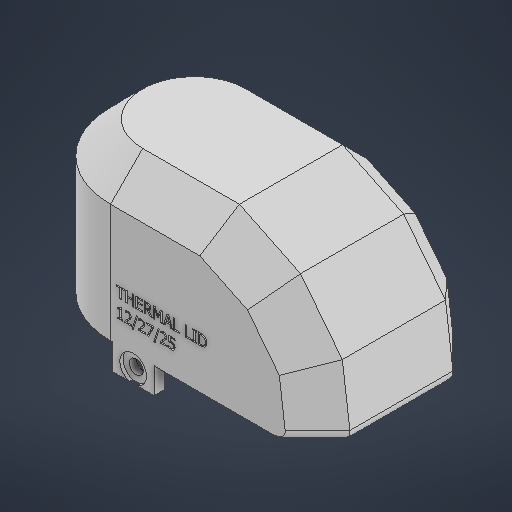
# Autodesk Inventor part: Thermal Lid
Saved by Autodesk Inventor 2026.2 (Build 302298000, 298)
## iProperties
Created: 2025-12-29
Part Number: Thermal Lid
Material: Generic
Document SubType Name: Modeling
Designer: mumin
Density: 1 g/cm^3
Appearance: Default
Author: mumin
Autodesk Inventor part; units mm, degrees
ref_plane "YZ Plane" through (0, 0, 0) normal (1, 0, 0) x (0, 1, 0)
ref_plane "XZ Plane" through (0, 0, 0) normal (0, 1, 0) x (-1, 0, 0)
ref_plane "XY Plane" through (0, 0, 0) normal (0, 0, 1) x (1, 0, 0)
sketch "Sketch1" plane through (0, 0, 0) normal (0, 0, 1) x (1, 0, 0)
  line L0 (0, 0) -> (0, 70)
  line L1 (0, 70) -> (84, 70)
  line L2 (84, 70) -> (112.4484, 56.2384)
  line L3 (112.4484, 56.2384) -> (131.9046, 31.3356)
  line L4 (131.9046, 31.3356) -> (136, 0)
  line L5 (-27.2, 0) -> (163.2, 0) projected
  line L6 (0, 0) -> (136, 0)
  dimension "d0" = 70
  dimension "d1" = 84
  dimension "d2" = 52
  dimension "d3" = 52
  constraints: 12 end point, 2 equal length, 1 collinear, 1 perpendicular, 1 point on line, 1 vertical
  measures "d0" distance of L0.start L0.end
  measures "d1" distance of L0.end L1.end
  measures "d2" horizontal distance of L1.end L4.end
  measures "d3" angle of L5 L3
extrude "Bilateral Extrude" add sketch "Sketch1" along normal mid plane 78
sketch "Sketch2" plane through (0, 70, -39) normal (0, 1, 0) x (1, 0, 0)
  line L0 (0, -39) -> (136, -39)
  line L1 (136, 0) -> (136, -78) projected
  line L2 (84, -78) -> (0, -78) projected
  arc A0 (39, 0) -> (39, -78) centre (39, -39) ccw
  line L3 (39, -39) -> (39, 0) construction
  line L4 (39, -39) -> (39, -78) construction
  line L5 (0, 0) -> (0, -78) projected
  line L6 (39, 0) -> (0, 0)
  line L7 (0, -78) -> (39, -78)
  dimension "d6" = 180
  constraints: 10 end point, 2 perpendicular, 2 point on circle, 2 point on line, 2 tangent, 1 centre point, 1 collinear, 1 midpoint
  measures "d6" angle of L3 L4
extrude "Rounded Front" cut sketch "Sketch2" against normal through all
shell "Shell1" thickness 5 removed faces 1 at (103.6667, 0, 13)
chamfer "Inside Chamfer" distance 12 angle 45 9 edges at (129.0406, 14.6667, 34) (118.174, 40.7886, 34) (96.0392, 58.6219, 34) (96.0392, 58.6219, -34) (118.174, 40.7886, -34) (129.0406, 14.6667, -34) (60.9271, 65, 34) (5, 65, 0) (60.9271, 65, -34)
chamfer "Outside Chamfer" distance 15 angle 45 9 edges at (61.5, 70, 39) (0, 70, 0) (61.5, 70, -39) (98.2242, 63.1192, 39) (98.2242, 63.1192, -39) (122.1765, 43.787, -39) (122.1765, 43.787, 39) (133.9523, 15.6678, 39) (133.9523, 15.6678, -39)
sketch "Sketch3" plane through (39, 0, 0) normal (0, -1, 0) x (1, 0, 0)
  line L0 (-39, -3.8185) -> (-39, 59.6275) construction
  line L1 (0.8, 39) -> (20.3, 39)
  line L2 (20.3, 39) -> (20.3, 34.2)
  line L3 (20.3, 34.2) -> (0.8, 34.2)
  line L4 (0.8, 34.2) -> (0.8, 39)
  line L5 (0, 39) -> (81.8724, 39) construction
  arc A0 (0, 39) -> (0, -39) centre (0, 0) ccw construction
  point P0 (-39, 0)
  point P1 (10.55, 39)
  dimension "d16" = 19.5
  dimension "d17" = 4.8
  dimension "d18" = 49.55
  constraints: 10 end point, 2 parallel, 1 horizontal, 1 midpoint, 1 perpendicular, 1 point on line, 1 tangent, 1 vertical
  measures "d16" distance of L2.end L3.end
  measures "d17" distance of L1.end L2.end
  measures "d18" distance from line of point (10.55, 39) L0
extrude "Alignment Tab" add sketch "Sketch3" along normal blind 12
sketch "Sketch4" plane through (0, 0, 39) normal (0, 0, 1) x (1, 0, 0)
  line L0 (49.55, -12) -> (49.55, 3)
  line L1 (59.3, -12) -> (39.8, -12) projected
  point P0 (0, 0)
  point P1 (49.55, -6)
  dimension "d28" = 15
  dimension "d29" = 6
  constraints: 2 end point, 1 point on line, 1 vertical
  measures "d28" distance of L0.start L0.end
  measures "d29" distance from line of L1 point (49.55, -6)
hole "Hole1" at (49.55, -6, 39) direction (0, 0, -1) diameter 6.5 depth 4.8 tip angle 118 counterbore diameter 12.5 counterbore depth 1.5
mirror "Mirror1" about plane through (0, 0, 0) normal (0, 0, 1) of "Alignment Tab", "Hole1"
sketch "Sketch6" plane through (0, 0, 39) normal (0, 0, 1) x (1, 0, 0)
  line L0 (41.5809, 23.9348) -> (84.0039, 23.9348) construction
  line L1 (84.0039, 23.9348) -> (84.0039, 9.6166) construction
  line L2 (84.0039, 9.6166) -> (41.5809, 9.6166) construction
  line L3 (41.5809, 9.6166) -> (41.5809, 23.9348) construction
  line L4 (43.2543, 18.9348) -> (43.2543, 23.3433)
  line L5 (43.2543, 23.3433) -> (41.5769, 23.3433)
  line L6 (41.5769, 23.3433) -> (41.5769, 23.9348)
  line L7 (41.5769, 23.9348) -> (45.5963, 23.9348)
  line L8 (45.5963, 23.9348) -> (45.5963, 23.3433)
  line L9 (45.5963, 23.3433) -> (43.9188, 23.3433)
  line L10 (43.9188, 23.3433) -> (43.9188, 18.9348)
  line L11 (43.9188, 18.9348) -> (43.2543, 18.9348)
  line L12 (49.7333, 18.9348) -> (49.0688, 18.9348)
  line L13 (49.0688, 18.9348) -> (49.0688, 21.3822)
  line L14 (49.0688, 21.3822) -> (46.7673, 21.3822)
  line L15 (46.7673, 21.3822) -> (46.7673, 18.9348)
  line L16 (46.7673, 18.9348) -> (46.1028, 18.9348)
  line L17 (46.1028, 18.9348) -> (46.1028, 23.9348)
  line L18 (46.1028, 23.9348) -> (46.7673, 23.9348)
  line L19 (46.7673, 23.9348) -> (46.7673, 21.9737)
  line L20 (46.7673, 21.9737) -> (49.0688, 21.9737)
  line L21 (49.0688, 21.9737) -> (49.0688, 23.9348)
  line L22 (49.0688, 23.9348) -> (49.7333, 23.9348)
  line L23 (49.7333, 23.9348) -> (49.7333, 18.9348)
  line L24 (50.7462, 18.9348) -> (50.7462, 23.9348)
  line L25 (50.7462, 23.9348) -> (53.8743, 23.9348)
  line L26 (53.8743, 23.9348) -> (53.8743, 23.3433)
  line L27 (53.8743, 23.3433) -> (51.4107, 23.3433)
  line L28 (51.4107, 23.3433) -> (51.4107, 21.9737)
  line L29 (51.4107, 21.9737) -> (53.7081, 21.9737)
  line L30 (53.7081, 21.9737) -> (53.7081, 21.3822)
  line L31 (53.7081, 21.3822) -> (51.4107, 21.3822)
  line L32 (51.4107, 21.3822) -> (51.4107, 19.5264)
  line L33 (51.4107, 19.5264) -> (53.8743, 19.5264)
  line L34 (53.8743, 19.5264) -> (53.8743, 18.9348)
  line L35 (53.8743, 18.9348) -> (50.7462, 18.9348)
  line L36 (58.4731, 18.9348) -> (57.6101, 18.9348)
  line L37 (57.6101, 18.9348) -> (56.0299, 20.9243)
  line L38 (56.0299, 20.9243) -> (55.2681, 20.9243)
  line L39 (55.2681, 20.9243) -> (55.2681, 18.9348)
  line L40 (55.2681, 18.9348) -> (54.6036, 18.9348)
  line L41 (54.6036, 18.9348) -> (54.6036, 23.9348)
  line L42 (54.6036, 23.9348) -> (55.8921, 23.9348)
  spline S0 degree 2 poles (55.8921, 23.9348) (56.3216, 23.9348) (56.901, 23.8416) (57.1644, 23.6715) knots 0 0 0 1 2 2 2
  spline S1 degree 2 poles (57.1644, 23.6715) (57.4278, 23.5013) (57.7316, 22.9705) (57.7316, 22.5775) knots 0 0 0 1 2 2 2
  spline S2 degree 2 poles (57.7316, 22.5775) (57.7316, 22.0305) (57.1725, 21.289) (56.6944, 21.1107) knots 0 0 0 1 2 2 2
  line L43 (56.6944, 21.1107) -> (58.4731, 18.9348)
  spline S3 degree 2 poles (57.0388, 22.5248) (57.0388, 22.7436) (56.8848, 23.0799) (56.7227, 23.1893) knots 0 0 0 1 2 2 2
  spline S4 degree 2 poles (56.7227, 23.1893) (56.5809, 23.2825) (56.2041, 23.3595) (55.9286, 23.3595) knots 0 0 0 1 2 2 2
  line L44 (55.9286, 23.3595) -> (55.2681, 23.3595)
  line L45 (55.2681, 23.3595) -> (55.2681, 21.4794)
  line L46 (55.2681, 21.4794) -> (55.8516, 21.4794)
  spline S5 degree 2 poles (55.8516, 21.4794) (56.1393, 21.4794) (56.5971, 21.5807) (56.7551, 21.7387) knots 0 0 0 1 2 2 2
  spline S6 degree 2 poles (56.7551, 21.7387) (56.901, 21.8765) (57.0388, 22.2655) (57.0388, 22.5248) knots 0 0 0 1 2 2 2
  line L47 (63.1571, 18.9348) -> (62.4926, 18.9348)
  line L48 (62.4926, 18.9348) -> (62.4926, 23.242)
  line L49 (62.4926, 23.242) -> (61.1879, 20.3125)
  line L50 (61.1879, 20.3125) -> (60.7827, 20.3125)
  line L51 (60.7827, 20.3125) -> (59.4902, 23.242)
  line L52 (59.4902, 23.242) -> (59.4902, 18.9348)
  line L53 (59.4902, 18.9348) -> (58.8702, 18.9348)
  line L54 (58.8702, 18.9348) -> (58.8702, 23.9348)
  line L55 (58.8702, 23.9348) -> (59.7778, 23.9348)
  line L56 (59.7778, 23.9348) -> (61.0258, 21.1512)
  line L57 (61.0258, 21.1512) -> (62.2333, 23.9348)
  line L58 (62.2333, 23.9348) -> (63.1571, 23.9348)
  line L59 (63.1571, 23.9348) -> (63.1571, 18.9348)
  line L60 (63.6312, 18.9348) -> (65.3167, 23.9348)
  line L61 (65.3167, 23.9348) -> (66.1352, 23.9348)
  line L62 (66.1352, 23.9348) -> (67.8208, 18.9348)
  line L63 (67.8208, 18.9348) -> (67.1198, 18.9348)
  line L64 (67.1198, 18.9348) -> (66.666, 20.3327)
  line L65 (66.666, 20.3327) -> (64.7576, 20.3327)
  line L66 (64.7576, 20.3327) -> (64.3038, 18.9348)
  line L67 (64.3038, 18.9348) -> (63.6312, 18.9348)
  line L68 (66.4837, 20.9) -> (65.7098, 23.2541)
  line L69 (65.7098, 23.2541) -> (64.9399, 20.9)
  line L70 (64.9399, 20.9) -> (66.4837, 20.9)
  line L71 (71.1919, 18.9348) -> (68.2949, 18.9348)
  line L72 (68.2949, 18.9348) -> (68.2949, 23.9348)
  line L73 (68.2949, 23.9348) -> (68.9594, 23.9348)
  line L74 (68.9594, 23.9348) -> (68.9594, 19.5264)
  line L75 (68.9594, 19.5264) -> (71.1919, 19.5264)
  line L76 (71.1919, 19.5264) -> (71.1919, 18.9348)
  line L77 (76.7592, 18.9348) -> (73.8621, 18.9348)
  line L78 (73.8621, 18.9348) -> (73.8621, 23.9348)
  line L79 (73.8621, 23.9348) -> (74.5266, 23.9348)
  line L80 (74.5266, 23.9348) -> (74.5266, 19.5264)
  line L81 (74.5266, 19.5264) -> (76.7592, 19.5264)
  line L82 (76.7592, 19.5264) -> (76.7592, 18.9348)
  line L83 (79.0242, 18.9348) -> (77.0874, 18.9348)
  line L84 (77.0874, 18.9348) -> (77.0874, 19.4454)
  line L85 (77.0874, 19.4454) -> (77.7235, 19.4454)
  line L86 (77.7235, 19.4454) -> (77.7235, 23.4243)
  line L87 (77.7235, 23.4243) -> (77.0874, 23.4243)
  line L88 (77.0874, 23.4243) -> (77.0874, 23.9348)
  line L89 (77.0874, 23.9348) -> (79.0242, 23.9348)
  line L90 (79.0242, 23.9348) -> (79.0242, 23.4243)
  line L91 (79.0242, 23.4243) -> (78.388, 23.4243)
  line L92 (78.388, 23.4243) -> (78.388, 19.4454)
  line L93 (78.388, 19.4454) -> (79.0242, 19.4454)
  line L94 (79.0242, 19.4454) -> (79.0242, 18.9348)
  spline S7 degree 2 poles (83.7892, 21.4308) (83.7892, 20.746) (83.2341, 19.6439) (82.7681, 19.336) knots 0 0 0 1 2 2 2
  spline S8 degree 2 poles (82.7681, 19.336) (82.3872, 19.0969) (81.6052, 18.9348) (80.9974, 18.9348) knots 0 0 0 1 2 2 2
  line L95 (80.9974, 18.9348) -> (79.8467, 18.9348)
  line L96 (79.8467, 18.9348) -> (79.8467, 23.9348)
  line L97 (79.8467, 23.9348) -> (80.9853, 23.9348)
  spline S9 degree 2 poles (80.9853, 23.9348) (81.6903, 23.9348) (82.4926, 23.7241) (82.7762, 23.5378) knots 0 0 0 1 2 2 2
  spline S10 degree 2 poles (82.7762, 23.5378) (83.2584, 23.2177) (83.7892, 22.1601) (83.7892, 21.4308) knots 0 0 0 1 2 2 2
  spline S11 degree 2 poles (83.0963, 21.4389) (83.0963, 22.0143) (82.7154, 22.8287) (82.3386, 23.0596) knots 0 0 0 1 2 2 2
  spline S12 degree 2 poles (82.3386, 23.0596) (82.0712, 23.2177) (81.4675, 23.3595) (81.0177, 23.3595) knots 0 0 0 1 2 2 2
  line L98 (81.0177, 23.3595) -> (80.5112, 23.3595)
  line L99 (80.5112, 23.3595) -> (80.5112, 19.5102)
  line L100 (80.5112, 19.5102) -> (81.0177, 19.5102)
  spline S13 degree 2 poles (81.0177, 19.5102) (81.4594, 19.5102) (82.1279, 19.652) (82.3994, 19.8425) knots 0 0 0 1 2 2 2
  spline S14 degree 2 poles (82.3994, 19.8425) (82.7479, 20.0775) (83.0963, 20.8554) (83.0963, 21.4389) knots 0 0 0 1 2 2 2
  line L101 (44.7778, 10.7025) -> (42.3386, 10.7025)
  line L102 (42.3386, 10.7025) -> (42.3386, 11.213)
  line L103 (42.3386, 11.213) -> (43.2462, 11.213)
  line L104 (43.2462, 11.213) -> (43.2462, 14.5639)
  line L105 (43.2462, 14.5639) -> (42.3386, 14.5639)
  line L106 (42.3386, 14.5639) -> (42.3386, 15.0218)
  spline S15 degree 2 poles (42.3386, 15.0218) (42.8532, 15.0218) (43.3394, 15.3135) (43.3718, 15.7187) knots 0 0 0 1 2 2 2
  line L107 (43.3718, 15.7187) -> (43.8905, 15.7187)
  line L108 (43.8905, 15.7187) -> (43.8905, 11.213)
  line L109 (43.8905, 11.213) -> (44.7778, 11.213)
  line L110 (44.7778, 11.213) -> (44.7778, 10.7025)
  line L111 (48.7811, 10.7025) -> (45.6976, 10.7025)
  line L112 (45.6976, 10.7025) -> (45.6976, 11.4115)
  spline S16 degree 2 poles (45.6976, 11.4115) (46.0299, 11.7235) (46.6214, 12.303) (46.9051, 12.615) knots 0 0 0 1 2 2 2
  spline S17 degree 2 poles (46.9051, 12.615) (47.4764, 13.243) (47.8937, 13.9966) (47.8937, 14.3978) knots 0 0 0 1 2 2 2
  spline S18 degree 2 poles (47.8937, 14.3978) (47.8937, 14.6085) (47.7641, 14.9245) (47.6466, 15.0258) knots 0 0 0 1 2 2 2
  spline S19 degree 2 poles (47.6466, 15.0258) (47.529, 15.1271) (47.2211, 15.2284) (47.0347, 15.2284) knots 0 0 0 1 2 2 2
  spline S20 degree 2 poles (47.0347, 15.2284) (46.8564, 15.2284) (46.4918, 15.1393) (46.3256, 15.0704) knots 0 0 0 1 2 2 2
  spline S21 degree 2 poles (46.3256, 15.0704) (46.1838, 15.0137) (45.9205, 14.8516) (45.8394, 14.7949) knots 0 0 0 1 2 2 2
  line L113 (45.8394, 14.7949) -> (45.803, 14.7949)
  line L114 (45.803, 14.7949) -> (45.803, 15.508)
  spline S22 degree 2 poles (45.803, 15.508) (46.0096, 15.6093) (46.7511, 15.8078) (47.0833, 15.8078) knots 0 0 0 1 2 2 2
  spline S23 degree 2 poles (47.0833, 15.8078) (47.7843, 15.8078) (48.5744, 15.0663) (48.5744, 14.4342) knots 0 0 0 1 2 2 2
  spline S24 degree 2 poles (48.5744, 14.4342) (48.5744, 14.1385) (48.4367, 13.6441) (48.3151, 13.4334) knots 0 0 0 1 2 2 2
  spline S25 degree 2 poles (48.3151, 13.4334) (48.1936, 13.2146) (47.841, 12.7851) (47.6466, 12.5785) knots 0 0 0 1 2 2 2
  spline S26 degree 2 poles (47.6466, 12.5785) (47.3305, 12.2341) (46.5566, 11.4966) (46.3256, 11.2819) knots 0 0 0 1 2 2 2
  line L115 (46.3256, 11.2819) -> (48.7811, 11.2819)
  line L116 (48.7811, 11.2819) -> (48.7811, 10.7025)
  line L117 (51.5282, 15.9253) -> (49.5712, 9.6166)
  line L118 (49.5712, 9.6166) -> (49.0039, 9.6166)
  line L119 (49.0039, 9.6166) -> (50.9529, 15.9253)
  line L120 (50.9529, 15.9253) -> (51.5282, 15.9253)
  line L121 (55.1628, 10.7025) -> (52.0793, 10.7025)
  line L122 (52.0793, 10.7025) -> (52.0793, 11.4115)
  spline S27 degree 2 poles (52.0793, 11.4115) (52.4115, 11.7235) (53.0031, 12.303) (53.2867, 12.615) knots 0 0 0 1 2 2 2
  spline S28 degree 2 poles (53.2867, 12.615) (53.8581, 13.243) (54.2754, 13.9966) (54.2754, 14.3978) knots 0 0 0 1 2 2 2
  spline S29 degree 2 poles (54.2754, 14.3978) (54.2754, 14.6085) (54.1457, 14.9245) (54.0282, 15.0258) knots 0 0 0 1 2 2 2
  spline S30 degree 2 poles (54.0282, 15.0258) (53.9107, 15.1271) (53.6028, 15.2284) (53.4164, 15.2284) knots 0 0 0 1 2 2 2
  spline S31 degree 2 poles (53.4164, 15.2284) (53.2381, 15.2284) (52.8735, 15.1393) (52.7073, 15.0704) knots 0 0 0 1 2 2 2
  spline S32 degree 2 poles (52.7073, 15.0704) (52.5655, 15.0137) (52.3021, 14.8516) (52.2211, 14.7949) knots 0 0 0 1 2 2 2
  line L123 (52.2211, 14.7949) -> (52.1846, 14.7949)
  line L124 (52.1846, 14.7949) -> (52.1846, 15.508)
  spline S33 degree 2 poles (52.1846, 15.508) (52.3913, 15.6093) (53.1328, 15.8078) (53.465, 15.8078) knots 0 0 0 1 2 2 2
  spline S34 degree 2 poles (53.465, 15.8078) (54.166, 15.8078) (54.9561, 15.0663) (54.9561, 14.4342) knots 0 0 0 1 2 2 2
  spline S35 degree 2 poles (54.9561, 14.4342) (54.9561, 14.1385) (54.8184, 13.6441) (54.6968, 13.4334) knots 0 0 0 1 2 2 2
  spline S36 degree 2 poles (54.6968, 13.4334) (54.5752, 13.2146) (54.2227, 12.7851) (54.0282, 12.5785) knots 0 0 0 1 2 2 2
  spline S37 degree 2 poles (54.0282, 12.5785) (53.7122, 12.2341) (52.9383, 11.4966) (52.7073, 11.2819) knots 0 0 0 1 2 2 2
  line L125 (52.7073, 11.2819) -> (55.1628, 11.2819)
  line L126 (55.1628, 11.2819) -> (55.1628, 10.7025)
  line L127 (58.9715, 14.9529) -> (56.8078, 10.7025)
  line L128 (56.8078, 10.7025) -> (56.0947, 10.7025)
  line L129 (56.0947, 10.7025) -> (58.3799, 15.115)
  line L130 (58.3799, 15.115) -> (55.7989, 15.115)
  line L131 (55.7989, 15.115) -> (55.7989, 15.7025)
  line L132 (55.7989, 15.7025) -> (58.9715, 15.7025)
  line L133 (58.9715, 15.7025) -> (58.9715, 14.9529)
  line L134 (61.662, 15.9253) -> (59.7049, 9.6166)
  line L135 (59.7049, 9.6166) -> (59.1376, 9.6166)
  line L136 (59.1376, 9.6166) -> (61.0866, 15.9253)
  line L137 (61.0866, 15.9253) -> (61.662, 15.9253)
  line L138 (65.2965, 10.7025) -> (62.213, 10.7025)
  line L139 (62.213, 10.7025) -> (62.213, 11.4115)
  spline S38 degree 2 poles (62.213, 11.4115) (62.5453, 11.7235) (63.1368, 12.303) (63.4205, 12.615) knots 0 0 0 1 2 2 2
  spline S39 degree 2 poles (63.4205, 12.615) (63.9918, 13.243) (64.4091, 13.9966) (64.4091, 14.3978) knots 0 0 0 1 2 2 2
  spline S40 degree 2 poles (64.4091, 14.3978) (64.4091, 14.6085) (64.2795, 14.9245) (64.162, 15.0258) knots 0 0 0 1 2 2 2
  spline S41 degree 2 poles (64.162, 15.0258) (64.0444, 15.1271) (63.7365, 15.2284) (63.5501, 15.2284) knots 0 0 0 1 2 2 2
  spline S42 degree 2 poles (63.5501, 15.2284) (63.3718, 15.2284) (63.0072, 15.1393) (62.841, 15.0704) knots 0 0 0 1 2 2 2
  spline S43 degree 2 poles (62.841, 15.0704) (62.6992, 15.0137) (62.4359, 14.8516) (62.3548, 14.7949) knots 0 0 0 1 2 2 2
  line L140 (62.3548, 14.7949) -> (62.3184, 14.7949)
  line L141 (62.3184, 14.7949) -> (62.3184, 15.508)
  spline S44 degree 2 poles (62.3184, 15.508) (62.525, 15.6093) (63.2665, 15.8078) (63.5987, 15.8078) knots 0 0 0 1 2 2 2
  spline S45 degree 2 poles (63.5987, 15.8078) (64.2997, 15.8078) (65.0898, 15.0663) (65.0898, 14.4342) knots 0 0 0 1 2 2 2
  spline S46 degree 2 poles (65.0898, 14.4342) (65.0898, 14.1385) (64.9521, 13.6441) (64.8305, 13.4334) knots 0 0 0 1 2 2 2
  spline S47 degree 2 poles (64.8305, 13.4334) (64.709, 13.2146) (64.3564, 12.7851) (64.162, 12.5785) knots 0 0 0 1 2 2 2
  spline S48 degree 2 poles (64.162, 12.5785) (63.8459, 12.2341) (63.072, 11.4966) (62.841, 11.2819) knots 0 0 0 1 2 2 2
  line L142 (62.841, 11.2819) -> (65.2965, 11.2819)
  line L143 (65.2965, 11.2819) -> (65.2965, 10.7025)
  spline S49 degree 2 poles (68.9958, 12.2908) (68.9958, 11.9302) (68.7649, 11.3143) (68.5542, 11.0874) knots 0 0 0 1 2 2 2
  spline S50 degree 2 poles (68.5542, 11.0874) (68.3435, 10.8605) (67.7154, 10.5971) (67.3265, 10.5971) knots 0 0 0 1 2 2 2
  spline S51 degree 2 poles (67.3265, 10.5971) (66.9699, 10.5971) (66.273, 10.7551) (66.0177, 10.8808) knots 0 0 0 1 2 2 2
  line L144 (66.0177, 10.8808) -> (66.0177, 11.5898)
  line L145 (66.0177, 11.5898) -> (66.0663, 11.5898)
  spline S52 degree 2 poles (66.0663, 11.5898) (66.1433, 11.5331) (66.431, 11.3872) (66.6052, 11.3224) knots 0 0 0 1 2 2 2
  spline S53 degree 2 poles (66.6052, 11.3224) (66.8038, 11.2535) (67.132, 11.1765) (67.3386, 11.1765) knots 0 0 0 1 2 2 2
  spline S54 degree 2 poles (67.3386, 11.1765) (67.5412, 11.1765) (67.9221, 11.3224) (68.0598, 11.4804) knots 0 0 0 1 2 2 2
  spline S55 degree 2 poles (68.0598, 11.4804) (68.1855, 11.6303) (68.3151, 12.0274) (68.3151, 12.2949) knots 0 0 0 1 2 2 2
  spline S56 degree 2 poles (68.3151, 12.2949) (68.3151, 12.5623) (68.1692, 12.9026) (68.0315, 13.0161) knots 0 0 0 1 2 2 2
  spline S57 degree 2 poles (68.0315, 13.0161) (67.8897, 13.1417) (67.4683, 13.247) (67.213, 13.247) knots 0 0 0 1 2 2 2
  spline S58 degree 2 poles (67.213, 13.247) (66.9375, 13.247) (66.3905, 13.162) (66.2243, 13.1255) knots 0 0 0 1 2 2 2
  line L146 (66.2243, 13.1255) -> (66.2243, 15.7025)
  line L147 (66.2243, 15.7025) -> (68.9675, 15.7025)
  line L148 (68.9675, 15.7025) -> (68.9675, 15.115)
  line L149 (68.9675, 15.115) -> (66.8686, 15.115)
  line L150 (66.8686, 15.115) -> (66.8686, 13.7819)
  spline S59 degree 2 poles (66.8686, 13.7819) (66.9902, 13.7981) (67.2252, 13.8103) (67.3224, 13.8103) knots 0 0 0 1 2 2 2
  spline S60 degree 2 poles (67.3224, 13.8103) (67.7073, 13.8103) (68.2381, 13.6846) (68.4812, 13.4983) knots 0 0 0 1 2 2 2
  spline S61 degree 2 poles (68.4812, 13.4983) (68.7284, 13.3119) (68.9958, 12.7446) (68.9958, 12.2908) knots 0 0 0 1 2 2 2
  point P0 (0, 0)
  dimension "d0" = 70
  dimension "d1" = 84
  dimension "d2" = 52
  dimension "d3" = 52
  constraints: 2 other
emboss "LABEL" sketch "Sketch6" operation cut depth 1 direction (0, 0, -1)
fillet "Fillet1" radius 4 3 edges at (128.4362, 0, 31.5) (136, 0, 0) (128.4362, 0, -31.5)
body "Solid1"
